Autodesk Inventor part; units mm, degrees
(part 6 of 6)
  line L2060 (-66.9703, -92.6564) -> (-81.1911, -92.6564) projected
  arc A219 (-84.9214, -91.5245) -> (-81.1911, -92.6564) centre (-81.1911, -85.944) ccw projected
  line L2061 (-84.9214, -91.5245) -> (-98.4236, -105.0267) projected
  line L2062 (-98.4236, -105.0267) -> (-76.5118, -126.9386) projected
  line L2063 (-76.5118, -126.9386) -> (-54.6, -105.0267) projected
  line L2064 (-54.6, -105.0267) -> (-66.9703, -92.6564) projected
  line L2065 (35.0455, -92.6564) -> (15.9624, -92.6564) projected
  line L2066 (15.9624, -92.6564) -> (3.5921, -105.0267) projected
  line L2067 (3.5921, -105.0267) -> (25.5039, -126.9386) projected
  line L2068 (25.5039, -126.9386) -> (47.4158, -105.0267) projected
  line L2069 (47.4158, -105.0267) -> (35.0455, -92.6564) projected
  line L2070 (59.7861, -92.6564) -> (42.2297, -92.6564) projected
  line L2071 (42.2297, -92.6564) -> (51.0079, -101.4346) projected
  line L2072 (51.0079, -101.4346) -> (59.7861, -92.6564) projected
  line L2073 (1.594, 93.8186) -> (0, 95.4126) projected
  line L2074 (0, 95.4126) -> (-1.594, 93.8186) projected
  line L2075 (-1.594, 93.8186) -> (1.594, 93.8186) projected
  line L2076 (42.2297, 93.8186) -> (47.4158, 99.0047) projected
  line L2077 (47.4158, 99.0047) -> (25.5039, 120.9165) projected
  line L2078 (25.5039, 120.9165) -> (3.5921, 99.0047) projected
  line L2079 (3.5921, 99.0047) -> (8.7782, 93.8186) projected
  line L2080 (8.7782, 93.8186) -> (42.2297, 93.8186) projected
  line L2081 (87.7843, 88.3654) -> (98.4236, 99.0047) projected
  line L2082 (98.4236, 99.0047) -> (76.5118, 120.9165) projected
  line L2083 (76.5118, 120.9165) -> (54.6, 99.0047) projected
  line L2084 (54.6, 99.0047) -> (59.7861, 93.8186) projected
  line L2085 (59.7861, 93.8186) -> (81.1911, 93.8186) projected
  arc A220 (87.7843, 88.3654) -> (81.1911, 93.8186) centre (81.1911, 87.1062) ccw projected
  line L2086 (87.9035, 65.7011) -> (102.0157, 51.5889) projected
  line L2087 (102.0157, 51.5889) -> (123.9275, 73.5007) projected
  line L2088 (123.9275, 73.5007) -> (102.0157, 95.4126) projected
  line L2089 (102.0157, 95.4126) -> (87.9035, 81.3004) projected
  line L2090 (87.9035, 81.3004) -> (87.9035, 65.7011) projected
  line L2091 (94.8078, 44.381) -> (98.4236, 47.9968) projected
  line L2092 (98.4236, 47.9968) -> (87.9035, 58.5169) projected
  line L2093 (87.9035, 58.5169) -> (87.9035, 54.9582) projected
  line L2094 (87.9035, 54.9582) -> (88.0954, 54.9582) projected
  arc A221 (94.8078, 48.2458) -> (88.0954, 54.9582) centre (88.0954, 48.2458) ccw projected
  line L2095 (94.8078, 48.2458) -> (94.8078, 44.381) projected
  line L2096 (94.8078, 7.789) -> (102.0157, 0.5811) projected
  line L2097 (102.0157, 0.5811) -> (123.9275, 22.4929) projected
  line L2098 (123.9275, 22.4929) -> (102.0157, 44.4047) projected
  line L2099 (102.0157, 44.4047) -> (94.8078, 37.1968) projected
  line L2100 (94.8078, 37.1968) -> (94.8078, 7.789) projected
  line L2101 (94.8078, -6.6269) -> (98.4236, -3.011) projected
  line L2102 (98.4236, -3.011) -> (94.8078, 0.6048) projected
  line L2103 (94.8078, 0.6048) -> (94.8078, -6.6269) projected
  line L2104 (94.8078, -43.2189) -> (102.0157, -50.4268) projected
  line L2105 (102.0157, -50.4268) -> (123.9275, -28.515) projected
  line L2106 (123.9275, -28.515) -> (102.0157, -6.6031) projected
  line L2107 (102.0157, -6.6031) -> (94.8078, -13.8111) projected
  line L2108 (94.8078, -13.8111) -> (94.8078, -43.2189) projected
  line L2109 (-87.9035, 81.3004) -> (-102.0157, 95.4126) projected
  line L2110 (-102.0157, 95.4126) -> (-123.9275, 73.5007) projected
  line L2111 (-123.9275, 73.5007) -> (-102.0157, 51.5889) projected
  line L2112 (-102.0157, 51.5889) -> (-87.9035, 65.7011) projected
  line L2113 (-87.9035, 65.7011) -> (-87.9035, 81.3004) projected
  line L2114 (-94.8078, 0.6048) -> (-98.4236, -3.011) projected
  line L2115 (-98.4236, -3.011) -> (-94.8078, -6.6269) projected
  line L2116 (-94.8078, -6.6269) -> (-94.8078, 0.6048) projected
  line L2117 (87.9035, -64.539) -> (98.4236, -54.0189) projected
  line L2118 (98.4236, -54.0189) -> (94.2247, -49.82) projected
  arc A222 (88.0954, -53.7961) -> (94.2247, -49.82) centre (88.0954, -47.0837) ccw projected
  line L2119 (88.0954, -53.7961) -> (87.9035, -53.7961) projected
  line L2120 (87.9035, -53.7961) -> (87.9035, -64.539) projected
  line L2121 (87.7843, -87.2033) -> (102.0157, -101.4346) projected
  line L2122 (102.0157, -101.4346) -> (123.9275, -79.5228) projected
  line L2123 (123.9275, -79.5228) -> (102.0157, -57.611) projected
  line L2124 (102.0157, -57.611) -> (87.9035, -71.7232) projected
  line L2125 (87.9035, -71.7232) -> (87.9035, -85.944) projected
  arc A223 (87.7843, -87.2033) -> (87.9035, -85.944) centre (81.1911, -85.944) ccw projected
  line L2126 (-8.7782, -92.6564) -> (0, -101.4346) projected
  line L2127 (0, -101.4346) -> (8.7782, -92.6564) projected
  line L2128 (8.7782, -92.6564) -> (-8.7782, -92.6564) projected
  line L2129 (-35.0455, -92.6564) -> (-47.4158, -105.0267) projected
  line L2130 (-47.4158, -105.0267) -> (-25.5039, -126.9386) projected
  line L2131 (-25.5039, -126.9386) -> (-3.5921, -105.0267) projected
  line L2132 (-3.5921, -105.0267) -> (-15.9624, -92.6564) projected
  line L2133 (-15.9624, -92.6564) -> (-35.0455, -92.6564) projected
  line L2134 (-59.7861, -92.6564) -> (-51.0079, -101.4346) projected
  line L2135 (-51.0079, -101.4346) -> (-42.2297, -92.6564) projected
  line L2136 (-42.2297, -92.6564) -> (-59.7861, -92.6564) projected
  line L2137 (66.9703, -92.6564) -> (54.6, -105.0267) projected
  line L2138 (54.6, -105.0267) -> (76.5118, -126.9386) projected
  line L2139 (76.5118, -126.9386) -> (98.4236, -105.0267) projected
  line L2140 (98.4236, -105.0267) -> (84.9214, -91.5245) projected
  arc A224 (81.1911, -92.6564) -> (84.9214, -91.5245) centre (81.1911, -85.944) ccw projected
  line L2141 (81.1911, -92.6564) -> (66.9703, -92.6564) projected
  line L2142 (-87.9035, -53.7961) -> (-87.9035, -64.539) projected
  line L2143 (81.1979, -102.0798) -> (81.1979, -102.0779)
  arc A225 (104.2312, 48.2458) -> (97.3269, 61.4799) centre (88.0954, 48.2458) ccw
  arc A226 (88.0954, 64.3816) -> (87.9035, 64.3804) centre (88.0954, 48.2458) ccw
  line L2144 (104.223, 44.3468) -> (104.2312, 44.381)
  point P0 (0, 0)
  point P1 (-87.9035, -92.6564)
  point P2 (94.8078, -53.7961)
  point P3 (-81.1979, 103.242)
  point P4 (87.9035, 64.3804)
  dimension "d128" = 6.7056
  dimension "d129" = 6.7056
  dimension "d130" = 6.7056
  dimension "d131" = 6.7056
  dimension "d132" = 6.7056
  dimension "d133" = 9.4234
  dimension "d134" = 9.4234
  dimension "d135" = 9.4234
  dimension "d136" = 9.4234
  dimension "d137" = 9.4234
  dimension "d138" = 9.4234
  dimension "d139" = 9.4234
  dimension "d140" = 9.4234
  dimension "d141" = 9.4234
  dimension "d142" = 9.4234
  constraints: 66 end point, 37 point on circle, 17 centre point, 13 point on line, 10 tangent, 7 vertical, 6 collinear, 5 parallel, 3 coincident, 3 horizontal, 2 equal radius, 2 midpoint, 1 perpendicular, 12 other
  measures "d128" radius of A2
  measures "d129" radius of A4
  measures "d130" radius of A5
  measures "d131" radius of A9
  measures "d132" radius of A10
  measures "d134" radial gap between concentric circles of A4 A11
  measures "d135" radial gap between concentric circles of A7 A14
  measures "d136" distance between parallel lines of L17 L39
  measures "d137" radial gap between concentric circles of A6 A15
  measures "d139" radial gap between concentric circles of A5 A16
  measures "d140" distance between parallel lines of L9 L41
  measures "d141" distance between parallel lines of L42 L43
  measures "d142" radial gap between concentric circles of A17 A18
extrude "Extrusion15" add sketch "Sketch14" against normal up to surface (3.175 mm away) contours L208 A11 L212 A4 | A0 L0 L225 L31 A11 L208 | L212 A11 L45 L316 L25 A4 | L225 L7 L217 L218 L216 L31 | L316 L45 A18 L328 L327 L11 A2 L319 L318 L25 | L216 L7 L145 L31 | L7 L218 L217 | L318 L319 A1 L12 L32 L25 | L145 L7 L144 L233 L123 L31 | A18 L43 L329 L330 L10 L327 L328 | L123 L7 L124 L31 | L124 L7 L107 L66 L64 L31 | L7 L233 L144 | L43 L323 L322 L15 L377 L376 L330 L329 | L64 L7 A10 L68 A12 L31 | L43 L324 L325 L15 L322 L323 | L7 L66 L107 | L43 L44 A19 L380 L379 L9 L333 L332 L15 L325 L324 | L68 A10 L70 A12 | L376 L377 L15 | L70 A10 L16 L74 L34 A12 | A19 L41 A16 L382 L9 L379 L380 | L332 L333 L9 L13 A3 L14 | L74 L16 L72 L373 A9 L22 L387 L386 A13 L34 | L386 L387 L18 L384 L385 L35 A13 | L16 L21 A8 L373 L72 | A16 L172 A5 L9 L382 | A16 L40 L339 L164 L8 A5 L172 | L385 L384 L22 L390 L389 L395 L394 L35 | L394 L395 L22 L392 L393 L35 | L40 L996 L995 L346 L152 L8 L195 L166 L164 L339 | L393 L392 L22 L400 L50 L17 L49 L404 A14 L38 L2144 L35 | L22 L389 L390 | L40 L995 L996 | L40 L347 L158 L8 L152 L346 | L166 L195 L8 | L19 A7 L20 L17 L50 L400 | L40 L550 L549 L413 L180 L8 L178 L162 L158 L347 | L404 L49 L3 L90 A15 L39 A14 | L40 L549 L550 | L40 L414 L92 L8 L180 L413 | L162 L178 L8 | L90 L5 A6 L88 A15 | L40 L945 L944 L408 L93 L8 L92 L414 | L88 A6 L6 L4 L93 L408 L40 A15 | L40 L944 L945
sketch "Sketch15" plane through (0, 3.175, 0) normal (0, 1, 0) x (1, 0, 0)
  line L0 (86.9474, -56.1232) -> (91.8331, -54.6192)
  line L1 (91.8331, -54.6192) -> (96.7682, -51.2034)
  line L2 (96.7682, -51.2034) -> (97.1041, -47.1687)
  line L3 (97.1041, -47.1687) -> (93.7619, -46.8905)
  line L4 (93.7619, -46.8905) -> (91.095, -50.622)
  line L5 (91.095, -50.622) -> (87.9034, -51.6044)
  line L6 (87.9034, -51.6044) -> (86.9474, -56.1232)
  line L7 (88.6358, -83.222) -> (85.6526, -87.396)
  line L8 (85.6526, -87.396) -> (83.0494, -91.0384)
  line L9 (83.0494, -91.0384) -> (79.56, -91.0384)
  line L10 (79.56, -91.0384) -> (78.5867, -95.6384)
  line L11 (78.5867, -95.6384) -> (84.3482, -94.4511)
  line L12 (84.3482, -94.4511) -> (89.9969, -91.5587)
  line L13 (89.9969, -91.5587) -> (91.5544, -85.3079)
  line L14 (91.5544, -85.3079) -> (88.6358, -83.222)
  line L15 (-88.4401, -84.4991) -> (-89.4119, -88.3991)
  line L16 (-89.4119, -88.3991) -> (-88.0075, -92.0574)
  arc A0 (-88.0075, -92.0574) -> (-87.3692, -92.9944) centre (-85.7004, -91.1717) ccw
  line L17 (-87.3692, -92.9944) -> (-83.4727, -93.9654)
  line L18 (-83.4727, -93.9654) -> (-78.8103, -93.4973)
  line L19 (-78.8103, -93.4973) -> (-80.5123, -91.0384)
  line L20 (-80.5123, -91.0384) -> (-84.4521, -89.6547)
  line L21 (-84.4521, -89.6547) -> (-86.4583, -86.7562)
  line L22 (-86.4583, -86.7562) -> (-86.7501, -83.8503)
  line L23 (-86.7501, -83.8503) -> (-88.4401, -84.4991)
  line L24 (-94.329, -47.6853) -> (-96.6545, -49.8944)
  line L25 (-96.6545, -49.8944) -> (-94.5696, -52.9066)
  line L26 (-94.5696, -52.9066) -> (-91.5291, -56.4797)
  line L27 (-91.5291, -56.4797) -> (-86.7391, -56.4797)
  line L28 (-86.7391, -56.4797) -> (-86.446, -52.9584)
  line L29 (-86.446, -52.9584) -> (-90.7584, -51.4439)
  line L30 (-90.7584, -51.4439) -> (-93.4165, -48.6458)
  line L31 (-93.4165, -48.6458) -> (-94.329, -47.6853)
  line L32 (-80.5557, 95.0843) -> (-84.5024, 94.271)
  line L33 (-84.5024, 94.271) -> (-88.6156, 92.692)
  line L34 (-88.6156, 92.692) -> (-89.2093, 91.0013)
  line L35 (-89.2093, 91.0013) -> (-90.3634, 87.7152)
  line L36 (-90.3634, 87.7152) -> (-88.6142, 85.8739)
  line L37 (-88.6142, 85.8739) -> (-86.609, 87.7788)
  line L38 (-86.609, 87.7788) -> (-85.3882, 88.9385)
  line L39 (-85.3882, 88.9385) -> (-82.7873, 91.4092)
  line L40 (-82.7873, 91.4092) -> (-81.4303, 91.6889)
  line L41 (-81.4303, 91.6889) -> (-80.2658, 92.136)
  line L42 (-80.2658, 92.136) -> (-79.8239, 94.2244)
  line L43 (-79.8239, 94.2244) -> (-80.5557, 95.0843)
  line L44 (80.5908, 94.9948) -> (84.4015, 94.9948)
  line L45 (84.4015, 94.9948) -> (87.4534, 93.4491)
  line L46 (87.4534, 93.4491) -> (88.4032, 90.975)
  line L47 (88.4032, 90.975) -> (89.266, 88.7275)
  line L48 (89.266, 88.7275) -> (88.1738, 86.5709)
  line L49 (88.1738, 86.5709) -> (86.6651, 87.6492)
  line L50 (86.6651, 87.6492) -> (86.114, 90.3239)
  line L51 (86.114, 90.3239) -> (84.2041, 91.6889)
  line L52 (84.2041, 91.6889) -> (81.6312, 92.5925)
  line L53 (81.6312, 92.5925) -> (78.957, 93.1583)
  line L54 (78.957, 93.1583) -> (79.8051, 94.8329)
  line L55 (79.8051, 94.8329) -> (80.5908, 94.9948)
  point P0 (0, 0)
  constraints: 112 end point, 18 parallel, 16 perpendicular, 10 point on line, 2 horizontal, 2 point on circle, 1 centre point, 1 collinear, 1 tangent
extrude "Extrusion16" add sketch "Sketch15" against normal up to surface (3.175 mm away)
sketch "Sketch17" plane through (0, 3.175, 0) normal (0, 1, 0) x (1, 0, 0)
  line L0 (-84.3661, -53.4337) -> (-84.3661, -85.944) projected
  line L1 (-84.3661, -69.6888) -> (-97.3269, -69.6888)
  line L2 (-97.3269, -85.9508) -> (-97.3269, -62.2998) projected
  circle A0 centre (-90.8465, -69.6888) radius 1.9939
  line L3 (-84.3661, 87.1062) -> (-84.3661, 54.5958) projected
  line L4 (-84.3661, 70.851) -> (-97.3269, 70.851)
  line L5 (-97.3269, 87.113) -> (-97.3269, 61.4799) projected
  circle A1 centre (-90.8465, 70.851) radius 1.9939
  line L6 (0, 374.7477) -> (0, -369.2956)
  line L7 (84.3661, -69.6888) -> (97.3269, -69.6888)
  circle A2 centre (90.8465, -69.6888) radius 1.9939
  line L8 (84.3661, 70.851) -> (97.3269, 70.851)
  circle A3 centre (90.8465, 70.851) radius 1.9939
  point P0 (0, 0)
  dimension "d149" = 3.9878
  dimension "d150" = 3.9878
  constraints: 10 end point, 6 symmetric about line, 4 centre point, 4 midpoint, 2 horizontal, 2 point on line, 1 vertical, 2 other
  measures "d149" diameter of A0
  measures "d150" diameter of A1
extrude "Extrusion17" cut sketch "Sketch17" against normal blind 55.5625
sketch "Sketch19" plane through (0, 3.175, 0) normal (0, 1, 0) x (1, 0, 0)
  line L0 (105.6078, -3.011) -> (127.5196, 18.9008) projected
  line L1 (127.5196, 18.9008) -> (149.4315, -3.011) projected
  line L2 (149.4315, -3.011) -> (127.5196, -24.9229) projected
  line L3 (127.5196, -24.9229) -> (105.6078, -3.011) projected
  circle A0 centre (127.5196, -3.011) radius 5.6261
  line L4 (121.0718, -11.7039) -> (117.6863, -15.0895)
  line L5 (118.8267, -9.4589) -> (115.4412, -12.8444)
  line L6 (136.2125, -9.4589) -> (139.5981, -12.8444)
  line L7 (133.9675, -11.7039) -> (137.353, -15.0895)
  line L8 (136.2125, 3.4368) -> (139.5981, 6.8223)
  line L9 (133.9675, 5.6818) -> (137.353, 9.0674)
  line L10 (121.0718, 5.6818) -> (117.6863, 9.0674)
  line L11 (118.8267, 3.4368) -> (115.4412, 6.8223)
  line L12 (118.8267, 3.4368) -> (118.9104, 3.3531)
  line L13 (121.0718, 5.6818) -> (121.1555, 5.5982)
  line L14 (134.2138, 5.9281) -> (133.8838, 5.5982)
  line L15 (136.3538, 3.578) -> (136.1288, 3.3531)
  line L16 (136.4385, -9.6848) -> (136.1288, -9.3752)
  line L17 (134.1934, -11.9299) -> (133.8838, -11.6202)
  line L18 (120.8459, -11.9299) -> (121.1555, -11.6202)
  line L19 (118.7191, -9.5665) -> (118.9104, -9.3752)
  arc A1 (118.9104, 3.3531) -> (118.9104, -9.3752) centre (127.5196, -3.011) ccw
  arc A2 (133.8838, 5.5982) -> (121.1555, 5.5982) centre (127.5196, -3.011) ccw
  arc A3 (121.1555, -11.6202) -> (133.8838, -11.6202) centre (127.5196, -3.011) ccw
  arc A4 (136.1288, -9.3752) -> (136.1288, 3.3531) centre (127.5196, -3.011) ccw
  point P0 (0, 0)
  dimension "d155" = 11.2522
  constraints: 32 end point, 8 point on circle, 6 point on line, 5 centre point
  measures "d155" diameter of A0
extrude "Extrusion19" add sketch "Sketch19" against normal up to surface (3.175 mm away) contours L0 L10 L13 A2 L14 L9 L1 L8 L15 A4 L16 L6 L2 L7 L17 A3 L18 L4 L3 L5 L19 A1 L12 L11
sketch "Sketch20" plane through (0, 3.175, 0) normal (0, 1, 0) x (1, 0, 0)
  line L0 (-28.5018, 125.9354) -> (28.1402, 125.9354)
  line L1 (28.1402, 125.9354) -> (28.1402, 152.6054)
  line L2 (28.1402, 152.6054) -> (-28.5018, 152.6054)
  line L3 (-28.5018, 152.6054) -> (-28.5018, 125.9354)
  line L4 (33.4391, 120.8554) -> (-33.8007, 120.8554)
  line L5 (-33.8007, 120.8554) -> (-33.8007, 157.6854)
  line L6 (-33.8007, 157.6854) -> (33.4391, 157.6854)
  line L7 (33.4391, 157.6854) -> (33.4391, 120.8554)
  line L8 (33.4391, 120.8554) -> (-33.8007, 157.6854) construction
  line L9 (-33.8007, 120.8554) -> (33.4391, 157.6854) construction
  circle A0 centre (-28.5018, 125.9354) radius 3.2639
  circle A1 centre (28.1402, 152.6054) radius 3.2639
  point P0 (0, 0)
  point P1 (-0.1808, 139.2704)
  dimension "d167" = 56.642
  dimension "d168" = 26.67
  dimension "d172" = 6.5278
  dimension "d173" = 6.5278
  dimension "d174" = 5.08
  dimension "d175" = 5.08
  constraints: 20 end point, 4 parallel, 2 centre point, 2 coincident, 2 horizontal, 2 midpoint, 2 perpendicular
  measures "d167" distance of L1.end L2.end
  measures "d168" distance of L2.end L0.start
  measures "d172" diameter of A0
  measures "d173" diameter of A1
  measures "d174" distance between parallel lines of L4 L0
  measures "d175" distance between parallel lines of L6 L2
extrude "Extrusion20" add sketch "Sketch20" against normal up to surface (3.175 mm away) contours A0 L3 L2 A1 L1 L0 | L4 L5 L6 L7
sketch "Sketch21" plane through (0, 3.175, 0) normal (0, 1, 0) x (1, 0, 0)
  line L0 (-33.8007, 120.8554) -> (33.4391, 120.8554)
  line L1 (33.4391, 120.8554) -> (33.4391, 157.6854)
  line L2 (33.4391, 157.6854) -> (-33.8007, 157.6854)
  line L3 (-33.8007, 157.6854) -> (-33.8007, 120.8554)
  circle A0 centre (28.1402, 152.6054) radius 3.2639 projected
  line L4 (28.1402, 152.6054) -> (28.1402, 125.9354)
  line L5 (28.1402, 125.9354) -> (-28.5018, 125.9354)
  circle A1 centre (-28.5018, 125.9354) radius 3.2639
  point P0 (0, 0)
  dimension "d180" = 26.67
  dimension "d181" = 56.642
  constraints: 12 end point, 2 parallel, 2 perpendicular, 1 centre point, 1 coincident, 1 horizontal, 1 vertical
  measures "d180" distance of L4.start L4.end
  measures "d181" distance of L4.end L5.end
extrude "Extrusion21" cut sketch "Sketch21" against normal blind 31.75 contours A1
body "Solid2"
